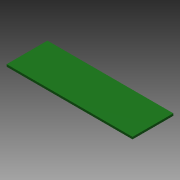
# Autodesk Inventor part: NoiseBoard
Saved by Autodesk Inventor 2014 (Build 180170000, 170)
## iProperties
Created: 2015-11-05
Part Number: NoiseBoard
Material: Generic
Document SubType Name: Modeling
Designer: Owner
Density: 1 g/cm^3
Appearance: Smooth - Dark Forest Green
Author: Owner
Autodesk Inventor part; units mm, degrees
ref_plane "YZ Plane" through (0, 0, 0) normal (1, 0, 0) x (0, 1, 0)
ref_plane "XZ Plane" through (0, 0, 0) normal (0, 1, 0) x (-1, 0, 0)
ref_plane "XY Plane" through (0, 0, 0) normal (0, 0, 1) x (1, 0, 0)
sketch "Sketch1" plane through (0, 0, 0) normal (0, 1, 0) x (-1, 0, 0)
  line L0 (-16.3083, 6.9019) -> (77.6717, 6.9019)
  line L1 (77.6717, 6.9019) -> (77.6717, -23.5781)
  line L2 (77.6717, -23.5781) -> (-16.3083, -23.5781)
  line L3 (-16.3083, -23.5781) -> (-16.3083, 6.9019)
  point P0 (0, 0)
  dimension "d0" = 93.98
  dimension "d1" = 30.48
  constraints: 8 end point, 2 parallel, 1 horizontal, 1 perpendicular
  measures "d0" distance of L0.start L0.end
  measures "d1" distance of L2.end L0.start
extrude "Extrusion1" add sketch "Sketch1" along normal blind 1.6
body "Solid1"
